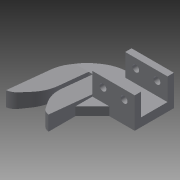
# Autodesk Inventor part: clip
Saved by Autodesk Inventor 2015 (Build 190159000, 159)
## iProperties
Created: 2017-12-17
Part Number: clip
Material: Generic
Document SubType Name: Modeling
Designer: Anshul
Density: 1 g/cm^3
Appearance: Default
Author: Anshul
Autodesk Inventor part; units mm, degrees
ref_plane "YZ Plane" through (0, 0, 0) normal (1, 0, 0) x (0, 1, 0)
ref_plane "XZ Plane" through (0, 0, 0) normal (0, 1, 0) x (-1, 0, 0)
ref_plane "XY Plane" through (0, 0, 0) normal (0, 0, 1) x (1, 0, 0)
sketch "Sketch1" plane through (0, 0, 0) normal (0, 1, 0) x (-1, 0, 0)
  line L0 (0, 0) -> (0, -12.5)
  line L1 (0, -12.5) -> (20, -12.5)
  line L2 (20, -12.5) -> (20, -15.5)
  line L3 (20, -15.5) -> (0, -15.5)
  line L4 (0, -15.5) -> (0, -12.5)
  line L5 (0, 0) -> (0, 3)
  line L6 (0, 3) -> (20, 3)
  line L7 (20, 3) -> (20, 0)
  line L8 (20, 0) -> (0, 0)
  line L9 (20, 0) -> (20, -12.5)
  line L10 (20, -6.25) -> (30, -6.25)
  line L11 (30, -6.25) -> (40, -6.25)
  line L12 (40, -6.25) -> (40, 23.75)
  line L13 (20, -6.25) -> (20, 23.75)
  line L14 (20, 23.75) -> (22, 23.75)
  line L15 (40, 23.75) -> (38, 23.75)
  line L16 (29, 13.75) -> (22, 23.75)
  line L17 (31, 13.75) -> (38, 23.75)
  line L18 (31, 13.75) -> (31, -6.25)
  line L19 (29, 13.75) -> (29, -6.25)
  line L20 (20, -15.5) -> (27, -15.5)
  line L21 (27, -15.5) -> (40, -6.25)
  line L22 (20, 3) -> (12, 3)
  line L23 (20, 3) -> (20, 11)
  line L24 (20, 11) -> (12, 3)
  line L25 (20, 3) -> (12, 3)
  line L26 (20, 3) -> (20, 11)
  dimension "d0" = 12.5
  dimension "d1" = 20
  dimension "d2" = 3
  dimension "d3" = 3
  dimension "d4" = 20
  dimension "d5" = 10
  dimension "d6" = 10
  dimension "d7" = 30
  dimension "d8" = 2
  dimension "d9" = 2
  dimension "d13" = 7
  dimension "d22" = 8
  dimension "d23" = 8
  constraints: 54 end point, 10 point on line, 8 perpendicular, 3 vertical, 2 horizontal, 1 collinear, 1 midpoint
  measures "d0" distance of L0.start L0.end
  measures "d1" distance of L0.end L1.end
  measures "d2" distance of L1.end L2.end
  measures "d3" distance of L0.start L5.end
  measures "d4" distance of L5.end L6.end
  measures "d5" distance of L10.start L10.end
  measures "d6" distance of L10.end L11.end
  measures "d7" distance of L11.end L12.end
  measures "d8" distance of L13.end L14.end
  measures "d9" distance of L12.end L15.end
  measures "d13" distance of L2.end L20.end
  measures "d22" distance of L6.end L22.end
  measures "d23" distance of L6.end L23.end
extrude "Extrusion1" add sketch "Sketch1" along normal blind 14.5 contours L5 L6 L7 L8 | L1 L2 L3 L4
extrude "Extrusion2" add sketch "Sketch1" along normal blind 4 contours L8 L9 L1 L0 | L9 L10 L11 L21 L20 L2
extrude "Extrusion3" add sketch "Sketch1" along normal blind 7 contours L7 L13 L14 L16 L19 L10 L9 | L11 L18 L17 L15 L12
sketch "Sketch2" plane through (-40, 0, -6.25) normal (-1, 0, 0) x (0, 0, 1)
  line L0 (6.25, 4) -> (-6.25, 4) projected
  line L1 (0, 4) -> (30, 7)
  line L2 (30, 7) -> (30, 0)
  line L3 (30, 0) -> (30, 7) projected
  line L4 (30, 0) -> (0, 0)
  line L5 (9.25, 0) -> (-9.25, 0) projected
  line L6 (0, 4) -> (0, 0)
  line L7 (0, 0) -> (0, 4) projected
  line L8 (0, 0) -> (0, 4)
  line L9 (0, 4) -> (0, 7) projected
  line L10 (0, 4) -> (0, 7)
  line L11 (0, 7) -> (30, 7)
  point P0 (6.25, 0)
  constraints: 14 end point, 3 collinear, 2 midpoint, 1 perpendicular, 1 vertical
extrude "Extrusion5" add sketch "Sketch1" along normal blind 4 contours L24 L13 L6
extrude "Extrusion6" cut sketch "Sketch2" against normal blind 20 contours L9 L11 L1
sketch "Sketch3" plane through (0, 14.5, -15.5) normal (0, 0, -1) x (-1, 0, 0)
  line L0 (20, 0) -> (0, 0)
  line L1 (0, 0) -> (20, 0) projected
  line L2 (10, 0) -> (20, 0)
  line L3 (15, 0) -> (15, -10.5)
  line L4 (20, -10.5) -> (12, -10.5) projected
  line L5 (15, -10.5) -> (15, -4.25)
  line L6 (10, 0) -> (0, 0)
  line L7 (5, 0) -> (5, -10.5)
  line L8 (0, -10.5) -> (20, -10.5) projected
  line L9 (5, -10.5) -> (5, -4.25)
  circle A0 centre (15, -4.25) radius 1.6
  circle A1 centre (5, -4.25) radius 1.6
  point P0 (0, -14.5)
  dimension "d28" = 6.25
  dimension "d29" = 6.25
  dimension "d30" = 3.2
  dimension "d31" = 3.2
  constraints: 14 end point, 4 point on line, 3 midpoint, 3 perpendicular, 2 centre point, 2 coincident, 1 collinear, 1 horizontal
  measures "d28" distance of L3.end L5.end
  measures "d29" distance of L7.end L9.end
  measures "d30" diameter of A0
  measures "d31" diameter of A1
extrude "Extrusion7" cut sketch "Sketch3" against normal blind 20 contours A0 L3 | L3 A0 | A1 L7 | L7 A1
fillet "Fillet1" radius 17 4 edges at (-31, 3, 13.75) (-29, 3, 13.75) (-27, 2, -15.5) (-40, 2, -6.25)
fillet "Fillet2" radius 5 2 edges at (-38, 3.5, 23.75) (-22, 3.5, 23.75)
body "Solid1"
